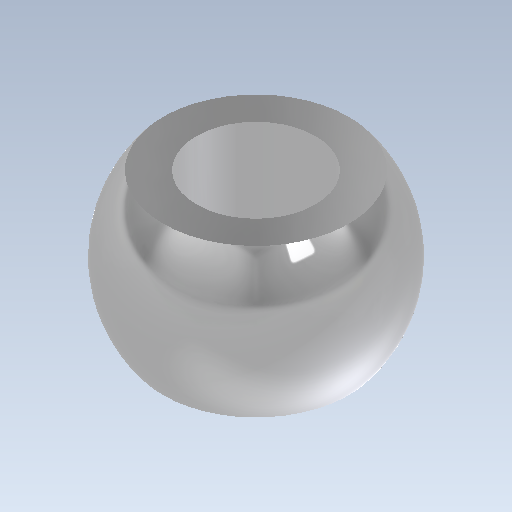
# Autodesk Inventor part: 500-109
Saved by Autodesk Inventor 2020 (Build 240168000, 168)
## iProperties
Created: 2015-04-18
Part Number: 500-109
Material: Aluminum 6061
Document SubType Name: Modeling
Designer: Station9
Density: 2.7 g/cm^3
Appearance: Aluminum - Flat
Mass: 0.215337 g
Surface Area: 1.43759 cm^2
Volume: 0.0797546 cm^3
Author: Station9
Autodesk Inventor part; units mm, degrees
ref_plane "YZ Plane" through (0, 0, 0) normal (1, 0, 0) x (0, 1, 0)
ref_plane "XZ Plane" through (0, 0, 0) normal (0, 1, 0) x (-1, 0, 0)
ref_plane "XY Plane" through (0, 0, 0) normal (0, 0, 1) x (1, 0, 0)
sketch "Sketch1" plane through (0, 0, 0) normal (0, 0, 1) x (1, 0, 0)
  arc A0 (0, -3.2) -> (0, 3.2) centre (0, 0) ccw
  line L0 (0, 3.2) -> (0, -3.2)
  dimension "d0" = 6.4
  constraints: 2 end point, 2 point on circle, 1 centre point, 1 coincident, 1 vertical
  measures "d0" diameter of A0
revolve "Revolution1" add sketch "Sketch1" angle 360 about axis through (0, 3.2, 0) along (0, -1, 0)
sketch "Sketch2" plane through (0, 0, 0) normal (1, 0, 0) x (0, 1, 0)
  line L0 (2, 8.8306) -> (-2, 8.8306)
  line L1 (-2, 8.8306) -> (-2, -8.8306)
  line L2 (-2, -8.8306) -> (2, -8.8306)
  line L3 (2, -8.8306) -> (2, 8.8306)
  line L4 (2, 8.8306) -> (-2, -8.8306) construction
  line L5 (-2, 8.8306) -> (2, -8.8306) construction
  line L6 (6.1175, 19.2226) -> (-9.7521, 19.2226)
  line L7 (-9.7521, 19.2226) -> (-9.7521, -16.6118)
  line L8 (-9.7521, -16.6118) -> (6.1175, -16.6118)
  line L9 (6.1175, -16.6118) -> (6.1175, 19.2226)
  point P0 (0, 0)
  dimension "d2" = 4
  constraints: 20 end point, 4 parallel, 2 horizontal, 2 midpoint, 2 perpendicular
  measures "d2" distance of L2.end L1.end
extrude "Extrusion1" cut sketch "Sketch2" along normal through all both and the other way through all
sketch "Sketch3" plane through (0, -2, 0) normal (0, -1, 0) x (1, 0, 0)
  circle A0 centre (0, 0) radius 2.498 projected
  circle A1 centre (0, 0) radius 1.6
  dimension "d5" = 3.2
  constraints: 1 centre point, 1 coincident
  measures "d5" diameter of A1
extrude "Extrusion2" cut sketch "Sketch3" against normal through all contours A1
body "Solid1"
